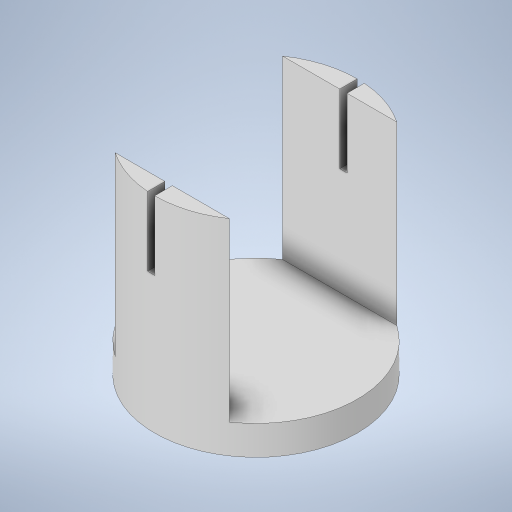
# Autodesk Inventor part: Base
Saved by Autodesk Inventor 2023 (Build 270158030, 158C)
## iProperties
Created: 2022-06-18
Part Number: Base
Material: Generic
Document SubType Name: Modeling
Designer: Mlees
Density: 1 g/cm^3
Appearance: Default
Author: Mlees
Autodesk Inventor part; units mm, degrees
ref_plane "YZ Plane" through (0, 0, 0) normal (1, 0, 0) x (0, 1, 0)
ref_plane "XZ Plane" through (0, 0, 0) normal (0, 1, 0) x (-1, 0, 0)
ref_plane "XY Plane" through (0, 0, 0) normal (0, 0, 1) x (1, 0, 0)
sketch "Sketch1" plane through (0, 0, 0) normal (1, 0, 0) x (0, 1, 0)
  circle A0 centre (0, -28.5) radius 34.5
  point P0 (0, 0)
  constraints: 1 centre point
extrude "Extrusion1" add sketch "Sketch1" along normal blind 70
sketch "Sketch2" plane through (70, 0, -28.5) normal (1, 0, 0) x (0, 0, -1)
  line L0 (-28.5, 0) -> (-28.5, 19.4422)
  circle A0 centre (0, 0) radius 34.5 projected
  line L1 (-28.5, 0) -> (-28.5, -19.4422)
  line L2 (28.5, 0) -> (28.5, 19.4422)
  line L3 (28.5, 0) -> (28.5, -19.4422)
  arc A1 (-28.5, 19.4422) -> (-28.5, -19.4422) centre (0, 0) ccw
  arc A2 (28.5, -19.4422) -> (28.5, 19.4422) centre (0, 0) ccw
  arc A3 (28.5, 19.4422) -> (-28.5, 19.4422) centre (0, 0) ccw
  arc A4 (-28.5, -19.4422) -> (28.5, -19.4422) centre (0, 0) ccw
  constraints: 12 point on circle, 8 end point, 6 concentric, 4 centre point, 2 point on line, 1 parallel, 1 vertical
extrude "Extrusion2" cut sketch "Sketch2" against normal blind 60 contours L0 A0 L2 L3 L1
sketch "Sketch3" plane through (70, 0, 0) normal (1, 0, 0) x (0, 0, -1)
  line L0 (0, 0) -> (0, 1.25)
  circle A0 centre (28.5, 0) radius 34.5 projected
  line L1 (28.5, 0) -> (28.5, 34.5)
  line L2 (0, 1.25) -> (0, 2.5)
  line L3 (0, -19.4422) -> (0, 19.4422) projected
  line L4 (0, 2.5) -> (-6.2328, 2.5)
  line L5 (-6.2328, 2.5) -> (-6.2328, 0)
  line L6 (-6.2328, 0) -> (0, 0)
  line L7 (57, 19.4422) -> (57, -19.4422) projected
  line L8 (57, 0) -> (57, -2.5)
  line L9 (57, -2.5) -> (63.7144, -2.5)
  line L10 (63.7144, -2.5) -> (63.7144, 0)
  line L11 (63.7144, 0) -> (57, 0)
  dimension "d9" = 1.25
  dimension "d10" = 2.5
  constraints: 20 end point, 6 perpendicular, 2 point on line, 1 midpoint, 1 point on circle, 1 vertical
  measures "d9" distance of L0.end L2.end
  measures "d10" distance of L8.start L8.end
extrude "Extrusion3" cut sketch "Sketch3" against normal blind 23.5 contours L6 A0 L4 L2 L0 | L6 L5 L4 A0 | L9 L7 L11 A0 | A0 L11 L10 L9
body "Solid1"
